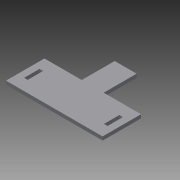
# Autodesk Inventor part: body-back
Saved by Autodesk Inventor 2013 (Build 170138000, 138)
## iProperties
Created: 2012-09-08
Part Number: body-back
Material: Generic
Document SubType Name: Modeling
Designer: frankenteddy
Density: 1 g/cm^3
Author: frankenteddy
Autodesk Inventor part; units mm, degrees
ref_plane "YZ Plane" through (0, 0, 0) normal (1, 0, 0) x (0, 1, 0)
ref_plane "XZ Plane" through (0, 0, 0) normal (0, 1, 0) x (-1, 0, 0)
ref_plane "XY Plane" through (0, 0, 0) normal (0, 0, 1) x (1, 0, 0)
sketch "Block1" plane through (0, 0, 0) normal (0, 0, 1) x (1, 0, 0)
  circle A0 centre (74.029, 24.2723) radius 1
  line L0 (49.279, 30.4723) -> (71.779, 30.4723)
  line L1 (71.779, 30.4723) -> (71.779, 18.0723)
  line L2 (71.779, 18.0723) -> (49.279, 18.0723)
  line L3 (49.279, 18.0723) -> (49.279, 30.4723)
  line L4 (49.279, 30.4723) -> (44.779, 30.4723)
  line L5 (44.779, 30.4723) -> (44.779, 18.0723)
  line L6 (44.779, 18.0723) -> (49.279, 18.0723)
  line L7 (49.279, 18.0723) -> (49.279, 30.4723)
  line L8 (71.779, 30.4723) -> (76.279, 30.4723)
  line L9 (76.279, 30.4723) -> (76.279, 18.0723)
  line L10 (76.279, 18.0723) -> (71.779, 18.0723)
  line L11 (71.779, 18.0723) -> (71.779, 30.4723)
  line L12 (44.779, 24.2723) -> (76.279, 24.2723) construction
  line L13 (47.029, 30.4723) -> (47.029, 18.0723) construction
  circle A1 centre (47.029, 24.2723) radius 1
  line L14 (74.029, 30.4723) -> (74.029, 18.0723) construction
  point P0 (60.979, 24.0984)
  dimension "d22" = 22.5
  dimension "d23" = 12.4
  dimension "d24" = 4.5
  dimension "d25" = 4.5
  dimension "d26" = 2
  dimension "d27" = 2
  measures "d22" distance of L1.end L2.end
  measures "d23" distance of L0.end L1.end
  measures "d24" distance of L6.end L5.end
  measures "d25" distance of L9.end L10.end
  measures "d26" diameter of A0
  measures "d27" diameter of A1
sketch "Sketch1" plane through (0, 0, 0) normal (0, 0, 1) x (1, 0, 0)
  line L0 (-50, 50) -> (50, 50)
  line L1 (50, 50) -> (50, -50)
  line L2 (50, -50) -> (-50, -50)
  line L3 (-50, -50) -> (-50, 50)
  line L4 (-92.7646, -8.503) -> (-89.7646, -8.503)
  line L5 (-89.7646, -8.503) -> (-89.7646, -11.753)
  line L6 (-89.7646, -11.753) -> (-92.7646, -11.753)
  line L7 (-92.7646, -11.753) -> (-92.7646, -8.503)
  line L8 (-92.7646, -21.6527) -> (-89.7646, -21.6527)
  line L9 (-89.7646, -21.6527) -> (-89.7646, -21.7527)
  line L10 (-89.7646, -21.7527) -> (-92.7646, -21.7527)
  line L11 (-92.7646, -21.7527) -> (-92.7646, -21.6527)
  line L12 (-50, 50) -> (-46.75, 50)
  line L13 (-46.75, 50) -> (-46.75, 36)
  line L14 (-46.75, 36) -> (-50, 36)
  line L15 (-50, 36) -> (-50, 50)
  line L16 (0, 50) -> (0, -50) construction
  line L17 (-50, 0) -> (50, 0) construction
  line L18 (50, 50) -> (46.75, 50)
  line L19 (46.75, 50) -> (46.75, 36)
  line L20 (46.75, 36) -> (50, 36)
  line L21 (50, 36) -> (50, 50)
  line L22 (-50, -50) -> (-46.75, -50)
  line L23 (-46.75, -50) -> (-46.75, -36)
  line L24 (-46.75, -36) -> (-50, -36)
  line L25 (-50, -36) -> (-50, -50)
  line L26 (46.75, -50) -> (46.75, -36)
  line L27 (46.75, -36) -> (50, -36)
  line L28 (50, -36) -> (50, -50)
  line L29 (50, -50) -> (46.75, -50)
  line L30 (-40, 40) -> (-10, 40)
  line L31 (-10, 40) -> (-10, 0)
  line L32 (-10, 0) -> (-40, 0)
  line L33 (-40, 0) -> (-40, 40)
  line L34 (40, 40) -> (10, 40)
  line L35 (10, 40) -> (10, 0)
  line L36 (10, 0) -> (40, 0)
  line L37 (40, 0) -> (40, 40)
  line L38 (-10, 50) -> (-6.75, 50)
  line L39 (-6.75, 50) -> (-6.75, 42)
  line L40 (-6.75, 42) -> (-10, 42)
  line L41 (-10, 42) -> (-10, 50)
  line L42 (10, 50) -> (6.75, 50)
  line L43 (6.75, 50) -> (6.75, 42)
  line L44 (6.75, 42) -> (10, 42)
  line L45 (10, 42) -> (10, 50)
  line L46 (-25, 0) -> (-25, 40) construction
  line L47 (-40, 50) -> (-43.25, 50)
  line L48 (-43.25, 50) -> (-43.25, 42)
  line L49 (-43.25, 42) -> (-40, 42)
  line L50 (-40, 42) -> (-40, 50)
  line L51 (43.25, 42) -> (40, 42)
  line L52 (43.25, 50) -> (43.25, 42)
  line L53 (40, 50) -> (43.25, 50)
  line L54 (40, 42) -> (40, 50)
  line L55 (0, -21.3) -> (0, -33.7) construction
  line L56 (-38, -16) -> (-34.75, -16)
  line L57 (-34.75, -16) -> (-34.75, -30)
  line L58 (-34.75, -30) -> (-38, -30)
  line L59 (-38, -30) -> (-38, -16)
  line L60 (-38, -23) -> (-34.75, -23) construction
  line L61 (38, -16) -> (34.75, -16)
  line L62 (34.75, -16) -> (34.75, -30)
  line L63 (34.75, -30) -> (38, -30)
  line L64 (38, -30) -> (38, -16)
  line L65 (38, -23) -> (34.75, -23) construction
  line L66 (-44, -40.5) -> (44, -40.5)
  line L67 (44, -40.5) -> (44, -5.5)
  line L68 (44, -5.5) -> (-44, -5.5)
  line L69 (-44, -5.5) -> (-44, -40.5)
  line L70 (-10, -5.5) -> (10, -5.5)
  line L71 (10, -5.5) -> (10, 24.5)
  line L72 (10, 24.5) -> (-10, 24.5)
  line L73 (-10, 24.5) -> (-10, -5.5)
  line L74 (44, -23) -> (-44, -23) construction
  point P0 (0, 0)
  dimension "d0" = 100
  dimension "d2" = 100
  dimension "d3" = 3
  dimension "mat" = 3.25
  dimension "d5" = 3
  dimension "kerf" = 0.1
  dimension "d7" = 3.25
  dimension "d8" = 14
  dimension "d9" = 30
  dimension "d10" = 40
  dimension "d11" = 10
  dimension "d12" = 10
  dimension "d15" = 3.25
  dimension "d16" = 8
  dimension "d17" = 0
  dimension "d28" = 22.5
  dimension "d29" = 3.25
  dimension "d30" = 14
  dimension "d31" = 12
  dimension "d34" = 6
  dimension "d35" = 6
  dimension "d38" = 20
  dimension "d39" = 30
  dimension "d42" = 35
  dimension "d43" = 9.5
  dimension "d44" = 20
  constraints: 150 end point, 31 symmetric about line, 18 parallel, 12 midpoint, 9 horizontal, 9 perpendicular, 3 point on line, 2 collinear, 2 other
  measures "d0" distance of L0.start L0.end
  measures "d2" distance of L2.end L0.start
  measures "d3" distance of L5.end L6.end
  measures "mat" distance of L4.end L5.end
  measures "d5" distance of L9.end L10.end
  measures "kerf" distance of L8.end L9.end
  measures "d7" distance of L13.end L14.end
  measures "d8" distance of L12.end L13.end
  measures "d9" distance of L31.end L32.end
  measures "d10" distance of L30.end L31.end
  measures "d11" distance between parallel lines of L30 L0
  measures "d12" distance between parallel lines of L3 L33
  measures "d15" distance of L39.end L40.end
  measures "d16" distance of L38.end L39.end
  measures "d17" distance between parallel lines of L41 L31
  measures "d29" distance of L57.end L58.end
  measures "d30" distance of L56.end L57.end
  measures "d31" distance between parallel lines of L59 L3
  measures "d34" distance between parallel lines of L59 L69
  measures "d35" distance between parallel lines of L67 L64
  measures "d38" distance between parallel lines of L71 L73
  measures "d39" distance between parallel lines of L70 L72
  measures "d42" distance between parallel lines of L66 L68
  measures "d43" distance between parallel lines of L2 L66
  measures "d44" distance between parallel lines of L2 L58
extrude "Extrusion5" add sketch "Sketch1" along normal blind 3.25 contours L72 L35 L71 L68 L73 L31 | L68 L67 L66 L69
equation "\"d7\" = mat"
equation "\"d15\" = mat"
equation "\"d29\" = mat"
equation "\"d40\" = mat"
body "Solid2"
